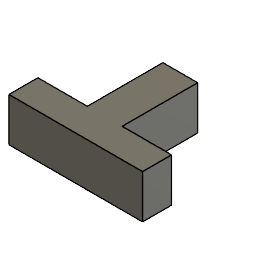
replay (Autodesk Fusion 360 design; units mm, degrees)
Autodesk Fusion 360 part; units mm, degrees
ref_plane "工作平面1" through (0, 20, 0) normal (0, 1, 0) x (0, 0, 1)
sketch "草图1" plane through (0, 20, 0) normal (0, 1, 0) x (1, 0, 0)
  line L0 (17, -35) -> (17, -9)
  line L1 (17, -9) -> (29, -9)
  line L2 (29, -9) -> (29, -35)
  line L3 (29, -35) -> (46, -35)
  line L4 (46, -35) -> (46, -45)
  line L5 (46, -45) -> (0, -45)
  line L6 (0, -45) -> (0, -35)
  line L7 (0, -35) -> (17, -35)
extrude "拉伸1" add sketch "草图1" against normal blind 15
